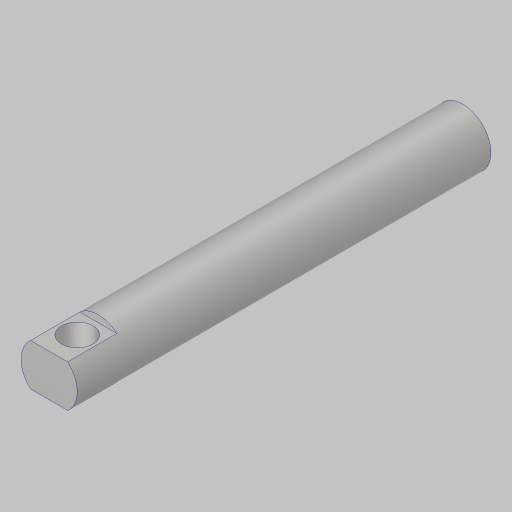
# Autodesk Inventor part: rod
Saved by Autodesk Inventor 2023.5 (Build 275446000, 446)
## iProperties
Created: 2025-01-30
Part Number: rod
Material: Aluminum 6061
Document SubType Name: Modeling
Designer: slick
Density: 2.7 g/cm^3
Appearance: Aluminum - Flat
Author: slick
Autodesk Inventor part; units mm, degrees
ref_plane "YZ Plane" through (0, 0, 0) normal (1, 0, 0) x (0, 1, 0)
ref_plane "XZ Plane" through (0, 0, 0) normal (0, 1, 0) x (-1, 0, 0)
ref_plane "XY Plane" through (0, 0, 0) normal (0, 0, 1) x (1, 0, 0)
sketch "Sketch1" plane through (0, 0, 0) normal (0, 0, 1) x (1, 0, 0)
  circle A0 centre (0, 0) radius 4
  dimension "d0" = 8
  constraints: 1 centre point, 1 coincident
  measures "d0" diameter of A0
extrude "Extrusion1" add sketch "Sketch1" along normal mid plane 59.0042
sketch "Sketch2" plane through (0, 0, 29.5021) normal (0, 0, 1) x (1, 0, 0)
  circle A0 centre (0, 0) radius 4 construction
  circle A1 centre (0, 0) radius 4 construction
  line L0 (-2.6458, 3) -> (2.6458, 3)
  line L1 (2.6458, -3) -> (-2.6458, -3)
  line L2 (0, 3) -> (0, -3) construction
  arc A2 (2.6458, 3) -> (-2.6458, 3) centre (0, 0) ccw
  arc A3 (-2.6458, -3) -> (2.6458, -3) centre (0, 0) ccw
  dimension "d3" = 6
  constraints: 8 point on circle, 6 end point, 3 coincident, 3 midpoint, 2 centre point, 1 horizontal, 1 parallel
  measures "d3" distance of L2.start L2.end
extrude "Extrusion2" cut sketch "Sketch2" against normal blind 7.0104
sketch "Sketch3" plane through (-2.6458, 3, 29.5021) normal (0, 1, 0) x (1, 0, 0)
  line L0 (5.2915, 7.0104) -> (0, 7.0104) construction
  point P0 (2.6458, 29.5021)
  point P1 (2.6458, 4.0104)
  point P2 (2.6458, 7.0104)
  dimension "d6" = 3
  constraints: 1 midpoint, 1 vertical alignment
  measures "d6" distance from line of L0 point (2.646, 4.01)
hole "Hole1" at (0, 3, 25.4917) direction (0, -1, 0) diameter 4.4958 end through all clearance for "Flat Head Machine Screw (82)" size "#8" standard "Ansi Unified Screw Threads"
body "Solid1"
